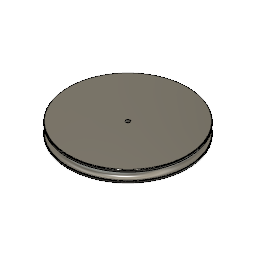
V1 (v4~recovered) (Autodesk Fusion 360 design; units mm, degrees)
Autodesk Fusion 360 part; units mm, degrees
note: some values were not read from the file. Chosen so that the rebuilt part matches the saved one: which face or edge a step refers to.
sketch "Sketch1" plane through (0, 0, 0) normal (0, 1, 0) x (1, 0, 0)
  circle A0 centre (0, 0) radius 18
  dimension "d1" = 36
  constraint coincident A0.centre origin
  measures "d1" diameter of A0
sketch "Sketch2" plane through (0, 0, 0) normal (0, 1, 0) x (1, 0, 0)
extrude "Extrude1" add sketch "Sketch1" along normal blind 50 makes body 1
sketch "Sketch3" plane through (0, 50, 0) normal (0, 1, 0) x (-1, 0, 0)
  circle A0 centre (0, 0) radius 18
  line L0 (-0.0027, -1.6) -> (0.0018, 1.05)
  line L1 (0.0018, 1.05) -> (-1.2055, 1.052)
  line L2 (0.0018, 1.05) -> (1.209, 1.048)
  arc A1 (-1.2055, 1.052) -> (1.209, 1.048) centre (0, 0) ccw
  circle A2 centre (0, 0) radius 1.6
  dimension "d7" = 3.2
  dimension "d9" = 2.65
  constraint coincident A0.centre A1.centre
  constraint coincident L0.start A1
  constraint perpendicular L0 L1
  constraint perpendicular L0 L2
  constraint concentric A1 A2
  constraint coincident L1.end A2
  measures "d7" diameter of A1
  measures "d9" distance of L0.start L0.end
extrude "Extrude2" add sketch "Sketch3" along normal blind 10 contours L0 L1 A1 A2 | L0 L2 A1 A2 bodies 1
sketch "Sketch1 (2)" plane through (0, 0, 0) normal (0, 1, 0) x (1, 0, 0) in component "SkjotariV3_PLA v6"
  circle A0 centre (0, 0) radius 60
  dimension "d1_1" = 120
  constraint coincident A0.centre origin
  measures "d1_1" diameter of A0
extrude "Extrude1'" add sketch "Sketch1 (2)" along normal blind 12 separate body makes body 2 in component "SkjotariV3_PLA v6"
sketch "Sketch2 (2)" plane through (0, 0, 0) normal (0, 0, 1) x (1, 0, 0) in component "SkjotariV3_PLA v6"
  line L0 (-60, 6) -> (-57.6, 6)
  arc A0 (-60.6, 3) -> (-60.6, 9) centre (-57.6, 6) ccw
  arc A1 (-60.6, 9) -> (-60.6, 3) centre (-57.6, 6) ccw
  constraint horizontal L0
  constraint coincident L0.end A0.centre
revolve "Revolve1" cut sketch "Sketch2 (2)" angle 360 about axis through (0, 0, 0) along (0, -1, 0) bodies 2 in component "SkjotariV3_PLA v6"
fillet "Fillet1" radius 0.3 1 edges at (-55.9396, 9.4986, 21.6969) on bodies 2 in component "SkjotariV3_PLA v6"
fillet "Fillet2" radius 0.3 1 edges at (-55.9396, 2.5014, -21.6969) on bodies 2 in component "SkjotariV3_PLA v6"
fillet "Fillet3" radius 0.5 1 edges at (-55.9396, 0, 21.6969) on bodies 2 in component "SkjotariV3_PLA v6"
fillet "Fillet4" radius 0.5 1 edges at (-55.9396, 12, 21.6969) on bodies 2 in component "SkjotariV3_PLA v6"
sketch "Sketch9" plane through (0, 87.336, 0) normal (0, 1, 0) x (-1, 0, 0)
  circle A0 centre (74.3311, -1.005) radius 59.5
  circle A1 centre (74.3311, -1.005) radius 1.95
  dimension "d61" = 3.9
  constraint concentric A0 A1
  measures "d61" diameter of A1
extrude "Extrude9" cut sketch "Sketch9" against normal blind 25 contours A1 sketch seen with x (1, 0, 0) y (0, 1, 0) z (0, 0, 1) at (74.3311, -75.336, 1.005) bodies 2 in component "SkjotariV3_PLA v6"
sketch "Sketch4" plane through (0, 12, 0) normal (0, 1, 0) x (-1, 0, 0) in component "SkjotariV3_PLA v6"
  circle A0 centre (0, 0) radius 59.5
  circle A1 centre (0, 0) radius 1.55
  circle A2 centre (0, 0) radius 59.5
  line L0 (24.3958, 12.8668) -> (35.4895, -15.766)
  line L1 (35.4895, -15.766) -> (31.388, -15.766)
  line L2 (31.388, -15.766) -> (23.9466, 5.0348)
  spline S0 degree 3 poles (23.9466, 5.0348) (23.6636, 5.8395) (23.1191, 7.3882) (22.6622, 8.9649) (22.4427, 9.7223) knots 0 0 0 0 0.25586 0.49237 0.49237 0.49237 0.49237
  spline S1 degree 3 poles (22.4427, 9.7223) (22.2114, 8.9384) (21.7456, 7.3599) (21.183, 5.8133) (20.8997, 5.0348) knots 0 0 0 0 0.24512 0.493597 0.493597 0.493597 0.493597
  line L3 (20.8997, 5.0348) -> (13.1653, -15.766)
  line L4 (13.1653, -15.766) -> (9.2981, -15.766)
  line L5 (9.2981, -15.766) -> (20.5091, 12.8668)
  line L6 (20.5091, 12.8668) -> (24.3958, 12.8668)
  spline S2 degree 3 poles (-18.665, -6.2627) (-18.7707, -6.2513) (-18.959, -6.2311) (-19.1483, -6.2259) (-19.2314, -6.2236) knots 0 0 0 0 0.031873 0.056795 0.056795 0.056795 0.056795
  spline S3 degree 5 poles (-59.1647, -9.9772) (-58.5704, -9.8764) (-57.4132, -9.6642) (-55.7708, -9.3139) (-53.7687, -8.7825) (-51.5831, -8.0102) (-49.7184, -7.1298) (-48.1765, -6.1434) (-46.9546, -5.0564) (-46.0423, -3.8794) (-45.4184, -2.6292) (-45.0583, -1.3277) (-44.9414, 0.0002) (-45.0584, 1.3281) (-45.4187, 2.6295) (-46.0426, 3.8796) (-46.9549, 5.0567) (-48.1767, 6.1438) (-49.7184, 7.1307) (-51.5829, 8.0118) (-53.7683, 8.7851) (-55.7701, 9.3174) (-57.4124, 9.6686) (-58.5696, 9.8815) (-59.1637, 9.9826) knots 0 0 0 0 0 0 0.05 0.1 0.15 0.2 0.25 0.3 0.35 0.4 0.45 0.5 0.55 0.6 0.65 0.7 0.75 0.8 0.85 0.9 0.95 1 1 1 1 1 1
  circle A3 centre (0, 0) radius 60
  line L7 (-59.1647, -9.9772) -> (-59.3128, -10.0023)
  line L8 (-59.1637, 9.9826) -> (-59.3461, 10.0136)
  line L9 (-21.8477, 12.9661) -> (-21.8477, 6.1106)
  line L10 (-21.8477, 6.1106) -> (-9.4258, 6.1106)
  line L11 (-9.4258, 6.1106) -> (-9.4258, 2.888)
  line L12 (-9.4258, 2.888) -> (-22.4922, -15.6667)
  line L13 (-22.4922, -15.6667) -> (-25.3633, -15.6667)
  line L14 (-25.3633, -15.6667) -> (-25.3633, 2.888)
  line L15 (-25.3633, 2.888) -> (-29.2305, 2.888)
  line L16 (-29.2305, 2.888) -> (-29.2305, 6.1106)
  line L17 (-29.2305, 6.1106) -> (-25.3633, 6.1106)
  line L18 (-25.3633, 6.1106) -> (-25.3633, 12.9661)
  line L19 (-25.3633, 12.9661) -> (-21.8477, 12.9661)
  line L20 (-21.8477, 2.888) -> (-21.8477, -10.0222)
  line L21 (-21.8477, -10.0222) -> (-12.8828, 2.888)
  line L22 (-12.8828, 2.888) -> (-21.8477, 2.888)
  point P0 (-47, -5)
  point P1 (-45, 0)
  point P2 (-47, 5)
  dimension "d11_1" = 3.1
  constraint concentric A0 A1
  constraint coincident S3.start A3
  constraint coincident S3.end A3
  measures "d11_1" diameter of A1
extrude "Extrude7" [suppressed] in component "SkjotariV3_PLA v6"
ref_plane "WorkPlane1" through (-0.4152, 6, 0.0022) normal (0, 1, 0) x (-1, 0, 0) in component "SkjotariV3_PLA v6"
mirror "Mirror2" [suppressed] in component "SkjotariV3_PLA v6"
extrude "Extrude5" [suppressed] in component "SkjotariV3_PLA v6"
extrude "Extrude8" [suppressed] in component "SkjotariV3_PLA v6"
extrude "Extrude3" [suppressed] in component "SkjotariV3_PLA v6"
extrude "Extrude4" [suppressed] in component "SkjotariV3_PLA v6"
sketch "Sketch6" plane through (0, 0, 0) normal (0, -1, 0) x (1, 0, 0) in component "SkjotariV3_PLA v6"
  circle A0 centre (0, 0) radius 1.55
  arc A1 (58.6712, 9.8966) -> (58.6721, -9.8914) centre (0, 0) ccw
  spline S0 degree 3 poles (58.6712, 9.8966) (56.0942, 9.4345) (52.3324, 8.5922) (48.1485, 6.1457) (47.2039, 5.3188) (45.8131, 3.5261) (45.4526, 2.6466) (45.0133, 1.0292) (44.9445, 0.0991) (45.1262, -1.5539) (45.344, -2.4957) (46.3784, -4.3665) (47.0387, -5.1192) (48.9464, -6.7158) (50.3173, -7.4352) (54.0966, -8.9739) (56.7187, -9.5423) (58.6721, -9.8914) knots 0.118723 0.118723 0.118723 0.118723 0.742092 0.742092 1.02193 1.02193 1.311544 1.311544 1.660435 1.660435 1.947559 1.947559 2.204945 2.204945 2.580611 2.580611 3.247512 3.247512 3.247512 3.247512
pattern_circular "C-Pattern1" [suppressed] in component "SkjotariV3_PLA v6"
fillet "Fillet5" [suppressed] in component "SkjotariV3_PLA v6"
fillet "Fillet6" [suppressed] in component "SkjotariV3_PLA v6"
fillet "Fillet7" [suppressed] in component "SkjotariV3_PLA v6"
fillet "Fillet8" [suppressed] in component "SkjotariV3_PLA v6"
sketch "Sketch4 (2)" plane through (0, 50, 0) normal (0, 1, 0) x (-1, 0, 0)
  arc A0 (-1.2055, 1.052) -> (1.209, 1.048) centre (0, 0) ccw
  line L0 (-1.2055, 1.052) -> (1.209, 1.048)
  circle A1 centre (0, 0) radius 18
  circle A2 centre (0, -10) radius 1.5
  circle A3 centre (8.6603, -5) radius 1.5
  circle A4 centre (8.6603, 5) radius 1.5
  circle A5 centre (0, 10) radius 1.5
  circle A6 centre (-8.6603, 5) radius 1.5
  circle A7 centre (-8.6603, -5) radius 1.5
  dimension "d18" = 3
  dimension "d20" = 360
  measures "d18" diameter of A2
extrude "Extrude3'" [suppressed]
sketch "Sketch5" plane through (0, 50, 0) normal (0, 1, 0) x (-1, 0, 0)
  circle A0 centre (-8.6603, 5) radius 1.5
  circle A1 centre (8.6603, -5) radius 1.5
  circle A2 centre (0, 10) radius 1.5
  circle A3 centre (-8.6603, -5) radius 1.5
  circle A4 centre (0, -10) radius 1.5
  circle A5 centre (8.6603, 5) radius 1.5
  arc A6 (-1.2055, 1.052) -> (1.209, 1.048) centre (0, 0) ccw
  line L0 (-1.2055, 1.052) -> (1.209, 1.048)
  circle A7 centre (0, 0) radius 18
  line L1 (-25, -25) -> (25, -25)
  line L2 (25, -25) -> (25, 25)
  line L3 (25, 25) -> (-25, 25)
  line L4 (-25, 25) -> (-25, -25)
  line L5 (-25, -25) -> (25, 25) construction
  line L6 (25, -25) -> (-25, 25) construction
  constraint horizontal L1
  constraint perpendicular L1 L2
  constraint parallel L1 L3
  constraint parallel L2 L4
  constraint coincident L5 A6.centre
  constraint coincident L6 A6.centre
  constraint coincident A6.centre A7.centre
extrude "Extrude4'" [suppressed]
sketch "Sketch6 (2)" plane through (0, 51, 0) normal (0, 1, 0) x (-1, 0, 0)
  circle A0 centre (0, -10) radius 1.5
  circle A1 centre (8.6603, 5) radius 1.5
  circle A2 centre (0, 10) radius 1.5
  circle A3 centre (-8.6603, -5) radius 1.5
  arc A4 (-1.2055, 1.052) -> (1.209, 1.048) centre (0, 0) ccw
  line L0 (-1.2055, 1.052) -> (1.209, 1.048)
  circle A5 centre (8.6603, -5) radius 1.5
  circle A6 centre (-8.6603, 5) radius 1.5
  line L1 (-25, 25) -> (-25, -25)
  line L2 (-25, -25) -> (25, -25)
  line L3 (25, -25) -> (25, 25)
  line L4 (25, 25) -> (-25, 25)
  circle A7 centre (20, -20) radius 1.5
  circle A8 centre (-20, -20) radius 1.5
  circle A9 centre (20, 20) radius 1.5
  circle A10 centre (-20, 20) radius 1.5
  dimension "d25" = 3
  dimension "d28" = -40
  dimension "d29" = 40
  measures "d25" diameter of A7
extrude "Extrude5'" [suppressed]
sketch "Sketch7" plane through (0, 51, 0) normal (0, 1, 0) x (-1, 0, 0)
  circle A0 centre (20, -20) radius 1.5
  circle A1 centre (-20, -20) radius 1.5
  circle A2 centre (20, 20) radius 1.5
  circle A3 centre (-20, 20) radius 1.5
  circle A4 centre (0, -10) radius 1.5
  arc A5 (-1.2055, 1.052) -> (1.209, 1.048) centre (0, 0) ccw
  line L0 (-1.2055, 1.052) -> (1.209, 1.048)
  circle A6 centre (-8.6603, -5) radius 1.5
  circle A7 centre (8.6603, 5) radius 1.5
  circle A8 centre (8.6603, -5) radius 1.5
  circle A9 centre (0, 10) radius 1.5
  circle A10 centre (-8.6603, 5) radius 1.5
  line L1 (-25, 25) -> (-25, -25)
  line L2 (-25, -25) -> (25, -25)
  line L3 (25, -25) -> (25, 25)
  line L4 (25, 25) -> (-25, 25)
  circle A11 centre (0, 0) radius 1.6
  constraint concentric A5 A11
  constraint coincident A5.start A11
extrude "Extrude6" [suppressed]
sketch "Sketch1 (3)" plane through (0, 0, 0) normal (0, 0, 1) x (1, 0, 0) in component "MjukurHringurSporoskjuMedGripi v6"
  line L0 (0, 0) -> (-55.1, 0)
  ellipse E0 centre (-55.1, 0) end of major axis (-55.1, 4.25) minor radius 5
  line L1 (-55.1, -4.25) -> (-55.1, 4.25)
  line L2 (-50.1, 0) -> (-60.1, 0)
  dimension "d1_2" = 55.1
  constraint coincident L0.start origin
  constraint horizontal L0
  constraint coincident L0.end E0.centre
  constraint coincident E0 L1.start
  constraint coincident E0 L1.end
  constraint coincident E0 L2.start
  constraint coincident E0 L2.end
  measures "d1_2" distance of L0.start L0.end
revolve "Revolve1'" [suppressed] in component "MjukurHringurSporoskjuMedGripi v6"
sketch "Sketch1 (4)" plane through (0, 0, 0) normal (0, 1, 0) x (1, 0, 0) in component "SkjotariV3_MjuktPlast v4"
  circle A0 centre (0, 0) radius 55
  dimension "d1_1_1" = 110
  constraint coincident A0.centre origin
  measures "d1_1_1" diameter of A0
sketch "Sketch2 (3)" plane through (0, 0, 0) normal (1, 0, 0) x (0, 0, -1) in component "SkjotariV3_MjuktPlast v4"
  circle A0 centre (-55.1185, 0) radius 4.25
  dimension "d2_1" = 8.5
  measures "d2_1" diameter of A0
revolve "Revolve1''" [suppressed] in component "SkjotariV3_MjuktPlast v4"
sketch "Sketch3 (2)" plane through (0, 0, 0) normal (0, 0, 1) x (1, 0, 0) in component "SkjotariV3_MjuktPlast v4"
ref_plane "WorkPlane2" through (0, -4, 0) normal (0, 1, 0) x (1, 0, 0) in component "SkjotariV3_MjuktPlast v4"
split "Split2" [suppressed] in component "SkjotariV3_MjuktPlast v4"
copy_body "Body->Comp1" [suppressed] in component "Component"
moveface "MoveFace1" [suppressed] in component "Component"
delete_face "DeleteFace1" [suppressed] in component "Component"
delete_face "DeleteFace2" [suppressed] in component "Component"
sketch "Sketch4 (3)" plane through (0, -4, 0) normal (0, 1, 0) x (1, 0, 0) in component "MjukurHringurSporoskjuMedGripi v6"
  spline S0 degree 5 poles (-59.5, 1) (-59.587, 0.98) (-59.7489, 0.94) (-59.9554, 0.88) (-60.1576, 0.8) (-60.2892, 0.7) (-60.3053, 0.6) (-60.2192, 0.5) (-60.0558, 0.4) (-59.8551, 0.3) (-59.6636, 0.2) (-59.5256, 0.1) (-59.4749, 0) (-59.5256, -0.1) (-59.6636, -0.2) (-59.8551, -0.3) (-60.0558, -0.4) (-60.2192, -0.5) (-60.3053, -0.6) (-60.2892, -0.7) (-60.1576, -0.8) (-59.9554, -0.88) (-59.7489, -0.94) (-59.587, -0.98) (-59.5, -1) knots 0 0 0 0 0 0 0.05 0.1 0.15 0.2 0.25 0.3 0.35 0.4 0.45 0.5 0.55 0.6 0.65 0.7 0.75 0.8 0.85 0.9 0.95 1 1 1 1 1 1
  line L0 (-60.2852, 0.6272) -> (-60.2852, -0.6375)
  line L1 (-50.1, 0) -> (-60.1, 0)
  circle A0 centre (0, 0) radius 50.1
  point P0 (-60.2, 0.5)
  point P1 (-59.5, 0)
  point P2 (-60.2, -0.5)
  constraint coincident S0 L0.start
  constraint coincident S0 L0.end
  constraint vertical L0
extrude "Extrude1''" [suppressed] in component "MjukurHringurSporoskjuMedGripi v6"
pattern_circular "C-Pattern2" [suppressed] in component "MjukurHringurSporoskjuMedGripi v6"
split "Split3" [suppressed] in component "MjukurHringurSporoskjuMedGripi v6"
moveface "MoveFace2" [suppressed] in component "MjukurHringurSporoskjuMedGripi v6"
delete_face "DeleteFace1'" [suppressed] in component "MjukurHringurSporoskjuMedGripi v6"
delete_face "DeleteFace2'" [suppressed] in component "MjukurHringurSporoskjuMedGripi v6"
move_body "Move1" [suppressed] in component "MjukurHringurSporoskjuMedGripi v6"
copy_body "CopyPasteBodies2" [suppressed]
move_body "Move2" [suppressed]
sketch "Sketch8" plane through (0, 60, 0) normal (0, 1, 0) x (-1, 0, 0)
  line L0 (-148.8331, 96.6381) -> (-144.9659, 96.6381)
  line L1 (-144.9659, 96.6381) -> (-144.9659, 103.4936)
  line L2 (-144.9659, 103.4936) -> (-141.4502, 103.4936)
  line L3 (-141.4502, 103.4936) -> (-141.4502, 96.6381)
  line L4 (-141.4502, 96.6381) -> (-129.0284, 96.6381)
  line L5 (-129.0284, 96.6381) -> (-129.0284, 93.4154)
  line L6 (-129.0284, 93.4154) -> (-142.0948, 74.8608)
  line L7 (-142.0948, 74.8608) -> (-144.9659, 74.8608)
  line L8 (-144.9659, 74.8608) -> (-144.9659, 93.4154)
  line L9 (-144.9659, 93.4154) -> (-148.8331, 93.4154)
  line L10 (-148.8331, 93.4154) -> (-148.8331, 96.6381)
  line L11 (-106.4373, 74.7615) -> (-110.3044, 74.7615)
  line L12 (-110.3044, 74.7615) -> (-99.0935, 103.3943)
  line L13 (-99.0935, 103.3943) -> (-95.2068, 103.3943)
  line L14 (-95.2068, 103.3943) -> (-84.113, 74.7615)
  line L15 (-84.113, 74.7615) -> (-88.2146, 74.7615)
  line L16 (-88.2146, 74.7615) -> (-95.656, 95.5622)
  spline S0 degree 3 poles (-95.656, 95.5622) (-95.939, 96.367) (-96.4834, 97.9157) (-96.9404, 99.4924) (-97.1599, 100.2497) knots 0 0 0 0 0.25586 0.49237 0.49237 0.49237 0.49237
  spline S1 degree 3 poles (-97.1599, 100.2497) (-97.3912, 99.4659) (-97.857, 97.8874) (-98.4196, 96.3408) (-98.7029, 95.5622) knots 0 0 0 0 0.24512 0.493597 0.493597 0.493597 0.493597
  line L17 (-98.7029, 95.5622) -> (-106.4373, 74.7615)
  circle A0 centre (-119.6026, 90.5275) radius 1.55
  spline S2 degree 3 poles (-178.1894, 80.1434) (-176.8237, 80.3874) (-175.4691, 80.6805) (-172.7973, 81.4233) (-171.4781, 81.872) (-169.2367, 82.9078) (-168.2897, 83.4442) (-166.5774, 84.7649) (-165.8152, 85.5564) (-164.4423, 87.7748) (-164.0478, 89.3183) (-164.1629, 92.192) (-164.5746, 93.5251) (-166.073, 95.8787) (-167.1808, 96.8559) (-169.5683, 98.3586) (-170.8399, 98.919) (-174.1052, 100.0763) (-176.1385, 100.5493) (-178.1885, 100.9167) knots -3.815244 -3.815244 -3.815244 -3.815244 -3.39903 -3.39903 -2.982815 -2.982815 -2.658412 -2.658412 -2.334008 -2.334008 -1.87594 -1.87594 -1.471204 -1.471204 -1.03898 -1.03898 -0.624815 -0.624815 0 0 0 0
  arc A1 (-178.1894, 80.1434) -> (-61.0166, 80.1382) centre (-119.6026, 90.5275) ccw
  spline S3 degree 3 poles (-61.0157, 100.9116) (-62.5014, 100.6461) (-63.9744, 100.323) (-66.8726, 99.4836) (-68.301, 98.9692) (-70.9413, 97.6163) (-72.1676, 96.7797) (-73.7637, 94.9735) (-74.2737, 94.1498) (-75.1582, 91.8031) (-75.2496, 90.1807) (-74.76, 88.1802) (-74.5914, 87.7023) (-73.7479, 85.9091) (-72.7157, 84.7876) (-70.7341, 83.3424) (-69.8777, 82.8652) (-67.5313, 81.7789) (-65.9915, 81.2808) (-63.305, 80.5849) (-62.1646, 80.344) (-61.0166, 80.1382) knots 0 0 0 0 0.452773 0.452773 0.905545 0.905545 1.342814 1.342814 1.628669 1.628669 2.095148 2.095148 2.246446 2.246446 2.689648 2.689648 2.982305 2.982305 3.465357 3.465357 3.815244 3.815244 3.815244 3.815244
  arc A2 (-61.0157, 100.9116) -> (-178.1885, 100.9167) centre (-119.6026, 90.5275) ccw
  circle A3 centre (-119.6026, 90.5275) radius 2
  dimension "d58" = 4
  constraint concentric A0 A3
  measures "d58" diameter of A3
extrude "Extrude7'" [suppressed]
component "SkjotariV3_PLA v6" placed x (1, 0, 0) y (0, 1, 0) z (0, 0, 1) at (0, 48, 0)
hidden bodies 1
equation "d1 = SkjótaraMótorBreidd"
equation "SkjótaraMótorBreidd = 36.0 mm"
equation "SkótaraMótorHæð = 50 mm"
equation "d4 = SkótaraMótorHæð"
equation "SkótaraMótorPinniBreidd = 3.2 mm"
equation "d7 = SkótaraMótorPinniBreidd"
equation "SkjótaraMótorPinniInnriBreidd = 2.65 mm"
equation "d9 = SkjótaraMótorPinniInnriBreidd"
named bodies: "SkjótaraMótorHægri", "SkjótaraMótorHægri (1)"
